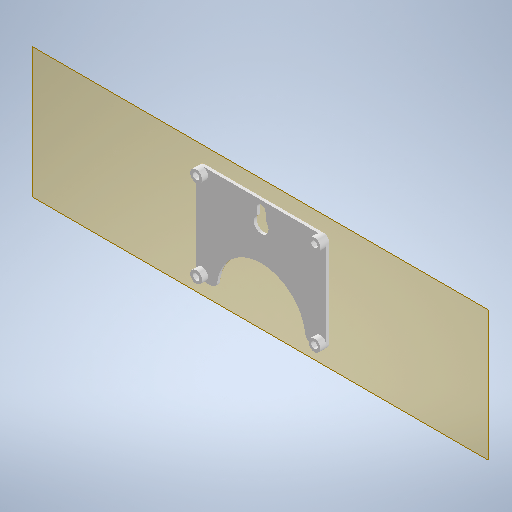
# Autodesk Inventor part: led 7 seg with sec v3 wall holder
Saved by Autodesk Inventor 2026 (Build 300175000, 175)
## iProperties
Created: 2025-08-20
Part Number: led 7 seg with sec v3 wall holder
Material: Generic
Document SubType Name: Modeling
Designer: Korobeynikov
Density: 1 g/cm^3
Appearance: Default
Author: Korobeynikov
Autodesk Inventor part; units mm, degrees
ref_plane "YZ Plane" through (0, 0, 0) normal (1, 0, 0) x (0, 1, 0)
ref_plane "XZ Plane" through (0, 0, 0) normal (0, 1, 0) x (-1, 0, 0)
ref_plane "XY Plane" through (0, 0, 0) normal (0, 0, 1) x (1, 0, 0)
ref_plane "Work Plane1" through (0, 0, 0) normal (0, 0, 1) x (1, 0, 0)
ref_plane "Work Plane2" through (0, 0, 0) normal (0, 0, 1) x (1, 0, 0)
sketch "Sketch2" plane through (0, 0, 0) normal (0, 0, 1) x (1, 0, 0)
  circle A0 centre (42.5, -29.5) radius 2.15 projected
  circle A1 centre (-37.5, -29.5) radius 2.15 projected
  circle A2 centre (-37.5, 29.5) radius 2.15 projected
  circle A3 centre (42.5, 29.5) radius 2.15 projected
  line L0 (-41.5, 33.5) -> (46.5, 33.5)
  line L1 (46.5, 33.5) -> (46.5, -33.5)
  line L2 (46.5, -33.5) -> (-41.5, -33.5)
  line L3 (-41.5, -33.5) -> (-41.5, 33.5)
  line L4 (-37.5, 29.5) -> (42.5, 29.5)
  point P0 (0, 0)
  point P1 (-41.5, 0)
  point P2 (2.5, 29.5)
  point P3 (2.5, 33.5)
  dimension "d0" = 67
  dimension "d1" = 88
  constraints: 10 end point, 3 midpoint, 2 horizontal, 2 parallel, 1 horizontal alignment, 1 perpendicular, 1 vertical alignment
  measures "d0" distance of L2.end L0.start
  measures "d1" distance of L0.start L0.end
extrude "Extrusion1" add sketch "Sketch2" along normal blind 2
sketch "Sketch3" plane through (0, 0, 2) normal (0, 0, 1) x (1, 0, 0)
  circle A0 centre (2.5, 18.7725) radius 5
  line L0 (46.5, 33.5) -> (-41.5, 33.5) projected
  circle A1 centre (2.5, 27.7153) radius 3
  line L1 (-0.5, 27.7153) -> (-0.5, 22.7725)
  line L2 (5.5, 27.7153) -> (5.5, 22.7725)
  point P0 (0, 0)
  point P1 (2.5, 33.5)
  dimension "d4" = 10
  dimension "d5" = 6
  constraints: 4 end point, 4 point on circle, 2 centre point, 2 tangent, 2 vertical alignment, 1 midpoint, 1 parallel, 1 vertical
  measures "d4" diameter of A0
  measures "d5" diameter of A1
extrude "Extrusion2" cut sketch "Sketch3" against normal through all
sketch "Sketch4" plane through (0, 0, 2) normal (0, 0, 1) x (1, 0, 0)
  circle A0 centre (-37.5, 29.5) radius 2.15 projected
  circle A1 centre (-37.5, 29.5) radius 4
  line L0 (46.5, 33.5) -> (-41.5, 33.5) projected
  circle A2 centre (-37.5, -29.5) radius 2.15 projected
  circle A3 centre (-37.5, -29.5) radius 4
  line L1 (-41.5, -33.5) -> (46.5, -33.5) projected
  circle A4 centre (42.5, -29.5) radius 2.15 projected
  circle A5 centre (42.5, -29.5) radius 4
  circle A6 centre (42.5, 29.5) radius 2.15 projected
  circle A7 centre (42.5, 29.5) radius 4
  point P0 (0, 0)
  constraints: 4 centre point, 4 coincident, 2 tangent
extrude "Extrusion3" add sketch "Sketch4" along normal blind 4
sketch "Sketch5" plane through (0, 0, 2) normal (0, 0, 1) x (1, 0, 0)
  line L0 (-41.5, -33.5) -> (46.5, -33.5) projected
  circle A0 centre (2.5, -33.5) radius 30
  point P0 (0, 0)
  point P1 (32.5, -33.5)
  point P2 (-27.5, -33.5)
  dimension "d10" = 60
  constraints: 1 centre point, 1 midpoint
  measures "d10" diameter of A0
extrude "Extrusion4" cut sketch "Sketch5" against normal through all contours A0 L0 picked at (9.9851, -22.0825)
fillet "Fillet1" radius 4 6 edges at (-41.5, 33.5, 1) (46.5, 33.5, 1) (-41.5, -33.5, 1) (46.5, -33.5, 1) (-27.5, -33.5, 1) (32.5, -33.5, 1)
body "Solid1"
